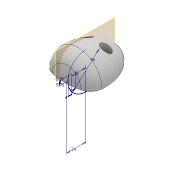
# Autodesk Inventor part: inner_body
Saved by Autodesk Inventor 2017 (Build 210142000, 142)
## iProperties
Created: 2018-06-30
Part Number: inner_body
Material: Generic
Document SubType Name: Modeling
Designer: mfans
Density: 1 g/cm^3
Appearance: Default
Author: mfans
Autodesk Inventor part; units mm, degrees
ref_plane "XZ Plane" through (0, 0, 0) normal (0, 1, 0) x (-1, 0, 0)
ref_plane "XY Plane" through (0, 0, 0) normal (0, 0, 1) x (1, 0, 0)
sketch "Sketch1" plane through (0, 0, 0) normal (0, 0, 1) x (1, 0, 0)
  line L0 (0, 0) -> (32, 0)
  line L1 (0, 0) -> (-32, 0)
  arc A0 (0, -6.678789) -> (32, 0) centre (0, 73.321211) ccw
  arc A1 (32, 0) -> (7.081838, 69.321211) centre (-26.517161, 18.104595) ccw
  line L2 (0, 69.321211) -> (0, -6.678789)
  line L3 (0, 69.321211) -> (7.081838, 69.321211)
  dimension "d0" = 32
  dimension "d1" = 32
  dimension "d2" = 80
  dimension "d3" = 4
  constraints: 8 end point, 4 point on circle, 3 horizontal, 2 centre point
  measures "d0" distance of L0.start L0.end
  measures "d1" distance of L0.start L1.end
  measures "d2" radius of A0
  measures "d3" distance from line of A0.centre L3
revolve "Revolution1" add sketch "Sketch1" angle 360 about axis through (0, 69.321211, 0) along (0, -1, 0)
fillet "Fillet1" radius 20 1 edges at (-32, 0, 0)
fillet "Fillet2" radius 20 1 edges at (-7.0818, 69.3212, 0)
thicken "Thicken1" operation add thickness 4 both sides no extend neighbours yes toward (-0.1644981, 0.9842195, 0.0652098) faces at (13.159851, -5.41635, -5.216785) (33.87103, 10.595478, 4.014803) (16.217696, 16.853217, -30.704008) (8.882006, 66.910275, -4.535394) (-0.155348, 69.321211, 0.046229)
sketch "Sketch2" plane through (0, 0, 0) normal (0, 0, 1) x (1, 0, 0)
  line L0 (-84.103756, 94.17302) -> (59.160517, 94.17302)
  line L1 (59.160517, 94.17302) -> (59.160517, -24.020002)
  line L2 (59.160517, -24.020002) -> (-84.103756, -24.020002)
  line L3 (-84.103756, -24.020002) -> (-84.103756, 94.17302)
  point P0 (0, 0)
  constraints: 8 end point, 2 parallel, 1 horizontal, 1 perpendicular
extrude "Extrusion1" cut sketch "Sketch2" against normal through all
sketch "Sketch3" plane through (0, 0, 0) normal (0, 0, 1) x (1, 0, 0)
  arc A0 (-18.530648, -0.385065) -> (18.530648, -0.385065) centre (0, 73.321211) ccw
  line L0 (0, -2.678789) -> (0, 37.321211)
  line L1 (0, 37.321211) -> (12, 37.321211)
  circle A1 centre (12, 37.321211) radius 6
  line L2 (0, 37.321211) -> (-12, 37.321211)
  circle A2 centre (-12, 37.321211) radius 6
  point P0 (0, 0)
  dimension "d11" = 40
  dimension "d12" = 12
  dimension "d13" = 12
  dimension "d14" = 12
  dimension "d15" = 12
  constraints: 6 end point, 2 centre point, 2 coincident, 1 horizontal, 1 perpendicular, 1 point on circle, 1 vertical
  measures "d11" distance of L0.start L0.end
  measures "d12" distance of L0.end L1.end
  measures "d13" diameter of A1
  measures "d14" distance of L0.end L2.end
  measures "d15" diameter of A2
extrude "Extrusion2" cut sketch "Sketch3" along normal through all
sketch "Sketch4" plane through (0, 0, 0) normal (1, 0, 0) x (0, 1, 0)
  arc A0 (47, 0) -> (24, 23) centre (24, 0) ccw
  line L0 (24, 0) -> (24, 23)
  line L1 (24, 0) -> (47, 0)
  line L2 (61.428343, 0) -> (13.979165, 0)
  circle A1 centre (24, 0) radius 23
  point P0 (0, 0)
  dimension "d18" = 46
  dimension "d19" = 24
  constraints: 4 end point, 2 centre point, 2 point on circle, 1 coincident, 1 point on line, 1 vertical
  measures "d18" diameter of A0
  measures "d19" distance of point (0, 0) L0.start
extrude "Extrusion3" cut sketch "Sketch4" along normal mid plane 38
sketch "Sketch5" plane through (0, 0, 0) normal (1, 0, 0) x (0, 1, 0)
  line L0 (47, 0) -> (1, 0)
  line L1 (24, 0) -> (6, 0)
  line L2 (6, 0) -> (6, 5.75)
  line L3 (6, 5.75) -> (24, 5.75)
  line L4 (24, 5.75) -> (24, 0)
  line L5 (6, 0) -> (2, 0)
  line L6 (2, 0) -> (2, 5.75)
  line L7 (2, 5.75) -> (6, 5.75)
  line L8 (6, 5.75) -> (6, 0)
  circle A0 centre (24, 0) radius 23
  line L9 (11, 5.75) -> (11, 18.973666)
  line L10 (11, 5.75) -> (11, 0)
  point P0 (0, 0)
  dimension "d22" = 5.75
  dimension "d23" = 18
  dimension "d24" = 4
  dimension "d25" = 5
  dimension "d26" = 5.75
  constraints: 20 end point, 4 parallel, 3 perpendicular, 2 horizontal, 2 point on line, 1 midpoint, 1 point on circle, 1 vertical
  measures "d22" distance between parallel lines of L0 L3
  measures "d23" distance of L2.end L3.end
  measures "d24" distance of L6.end L7.end
  measures "d25" distance between parallel lines of L2 L9
  measures "d26" distance of L5.end L6.end
extrude "Extrusion4" add sketch "Sketch5" along normal up to surface (38 mm away) from surface at -19 contours L9 L3 L7 L6 L0 A0 | L0 L2 L3 L10 | L6 L7 L2 L0
ref_plane "Work Plane1" through (-8, 0, 0) normal (1, 0, 0) x (0, 1, 0)
sketch "Sketch6" plane through (-8, 0, 0) normal (1, 0, 0) x (0, 1, 0)
  line L0 (11, 5.75) -> (11, 0)
  line L1 (47, 0) -> (1, 0)
  line L2 (6, 5.75) -> (6, 0)
  line L3 (24, 0) -> (6, 0)
  line L4 (11, 5.140513) -> (6, 5.140513)
  point P0 (0, 0)
  constraints: 2 end point, 2 point on line, 1 perpendicular
extrude "Extrusion5" cut sketch "Sketch6" against normal blind 20.5
body "Solid1"
